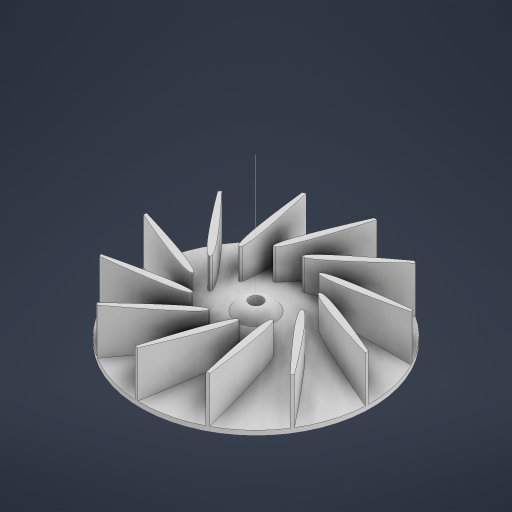
# Autodesk Inventor part: FanWing_open
Saved by Autodesk Inventor 2023 (Build 270158000, 158)
## iProperties
Created: 2023-02-14
Part Number: FanWing_open
Material: 一般
Document SubType Name: Modeling
Designer: neko2
Density: 1 g/cm^3
Appearance: 既定
Author: neko2
Autodesk Inventor part; units mm, degrees
ref_plane "YZ Plane" through (0, 0, 0) normal (1, 0, 0) x (0, 1, 0)
ref_plane "XZ Plane" through (0, 0, 0) normal (0, 1, 0) x (-1, 0, 0)
ref_plane "XY Plane" through (0, 0, 0) normal (0, 0, 1) x (1, 0, 0)
sketch "スケッチ1" plane through (0, 0, 0) normal (0, 1, 0) x (-1, 0, 0)
  circle A0 centre (0, 0) radius 7.5
  dimension "d0" = 15
  constraints: 1 centre point, 1 coincident
  measures "d0" diameter of A0
extrude "押し出し1" add sketch "スケッチ1" along normal blind 0.3
sketch "スケッチ2" plane through (0, 0.3, 0) normal (0, 1, 0) x (1, 0, 0)
  circle A0 centre (0, 0) radius 7.5 projected
  line L0 (-3, 0) -> (-6.3495, 3.9918)
  line L1 (-3, 0) -> (-3, 2.578)
  line L2 (0, 0) -> (-7.5, 0)
  line L3 (-3, 0) -> (-2.7429, 0.3064) construction
  line L4 (-2.7429, 0.3064) -> (-6.2979, 4.0726) construction
  spline S0 degree 2 poles (-3, 0) (-2.7429, 0.3064) (-6.2979, 4.0726) knots 1 1 1 2 2 2
  circle A1 centre (0, 0) radius 7.5 projected
  line L5 (-6.2979, 4.0726) -> (-3, 0)
  line L6 (-2.7429, 0.3064) -> (-3, 0)
  spline S1 degree 2 poles (-3, 0) (-3.3464, -0.2) (-6.4381, 3.955) knots 1 1 1 2 2 2
  line L7 (-3, 0) -> (-3.3464, -0.2) construction
  line L8 (-3.3464, -0.2) -> (-6.4381, 3.955) construction
  point P0 (-3, 0.1456)
  point P1 (-6.4021, 3.9068)
  point P2 (-3.0868, 0)
  dimension "d22" = 40
  dimension "d25" = 3
  dimension "d40" = 1
  dimension "d41" = 80
  dimension "d42" = 0.4
  constraints: 10 end point, 3 point on circle, 2 symmetric about line, 1 coincident, 1 horizontal, 1 point on line, 1 vertical, 6 other
  measures "d22" angle of L1 L0
  measures "d25" distance of point (0, 0) L0.start
  measures "d40" angle of L5 L0
  measures "d41" angle of L0 L3
  measures "d42" distance of L0.start L3.end
extrude "押し出し2" add sketch "スケッチ2" along normal blind 3 contours L5 L0 A0 | S0 L1 L5 | L0 L2 S1 A0 | S0 L1
pattern_circular "円形状パターン1" count 12 over 360 about axis through (0, 0, 0) along (0, 1, 0) of "押し出し2"
sketch "スケッチ11" plane through (0, 0, 0) normal (0, 0, 1) x (1, 0, 0)
  line L0 (7.5, 0) -> (-7.5, 0) projected
  line L1 (-7.5, 0) -> (-7.5, 4.832)
  line L2 (-7.5, 0) -> (-7.5, 0.3) projected
  line L3 (-6.6759, 0.3) -> (-7.5, 0.3) projected
  line L4 (-7.5, 0.3) -> (0, 2)
  line L5 (0, -0.9664) -> (0, 5.7984) projected
  point P0 (0, 0)
  point P1 (-7.4978, 0.3)
  dimension "d44" = 2
  constraints: 4 end point, 1 collinear, 1 point on line
  measures "d44" distance of point (0, 0) L4.end
revolve "回転6" add sketch "スケッチ11" angle 360 about axis through (0, 0, 0) along (0, 1, 0)
sketch "スケッチ3" plane through (0, 0.3, 0) normal (0, 1, 0) x (1, 0, 0)
  circle A0 centre (0, 0) radius 1.25
  dimension "d17" = 2.5
  constraints: 1 centre point, 1 coincident
  measures "d17" diameter of A0
extrude "押し出し3" add sketch "スケッチ3" along normal blind 2
sketch "スケッチ4" plane through (0, 2.3, 0) normal (0, 1, 0) x (1, 0, 0)
  circle A0 centre (0, 0) radius 0.425
  dimension "d21" = 0.85
  constraints: 1 centre point, 1 coincident
  measures "d21" diameter of A0
extrude "押し出し4" cut sketch "スケッチ4" against normal through all
fillet "フィレット5" radius 1 1 edges at (-1.25, 2.3, 0)
